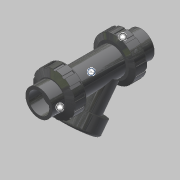
# Autodesk Inventor part: STRAINER Y-TYPE GLUED DN40
Saved by Autodesk Inventor 2017 (Build 210142000, 142)
## iProperties
Company: Pocket Brewery Belgium
Created: 2016-04-26
Part Number: STRAINER Y-TYPE GLUED DN40
Description: RVUIV VINK
Document SubType Name: Modeling
Manufacturer: SEKISUI
Mass: 197.859 g
Surface Area: 285.44 cm^2
Volume: 153.379 cm^3
Density: 1.29 g/cm^3
Material: U-PVC
Appearance: Smooth - Medium Gray
Catalog Web Link: http://www.pocketbrewery.com
Title: BALL VALVE PVC-U TRD DN15
Autodesk Inventor part; units mm, degrees
ref_plane "YZ Plane" through (0, 0, 0) normal (1, 0, 0) x (0, 1, 0)
ref_plane "XZ Plane" through (0, 0, 0) normal (0, 1, 0) x (-1, 0, 0)
ref_plane "XY Plane" through (0, 0, 0) normal (0, 0, 1) x (1, 0, 0)
sketch "Sketch_1" plane through (0, 0, 0) normal (1, 0, 0) x (0, 1, 0)
  line L0 (90.5, 0) -> (90.5, -33.3333)
  line L1 (90.5, -33.3333) -> (84.4338, -50)
  line L2 (84.4338, -50) -> (58.7082, -50)
  line L3 (58.7082, -50) -> (54.3, -37.8886)
  line L4 (54.3, -37.8886) -> (54.3, -25)
  line L5 (-54.3, -25) -> (-54.3, -37.8886)
  line L6 (-54.3, -37.8886) -> (-58.7082, -50)
  line L7 (-58.7082, -50) -> (-84.4338, -50)
  line L8 (-84.4338, -50) -> (-90.5, -33.3333)
  line L9 (-90.5, -33.3333) -> (-90.5, 0)
  line L10 (-90.5, 0) -> (90.5, 0)
  line L11 (-58.7082, -50) -> (0, -50) construction
  line L12 (0, -50) -> (0, -44.4444) construction
  line L13 (-85.1618, -50) -> (-60.7082, -50)
  line L14 (-60.7082, -50) -> (-60.7082, -48)
  line L15 (-60.7082, -48) -> (-85.1618, -48)
  line L16 (-85.1618, -48) -> (-85.1618, -50)
  line L17 (60.7082, -50) -> (85.1618, -50)
  line L18 (85.1618, -50) -> (85.1618, -48)
  line L19 (85.1618, -48) -> (60.7082, -48)
  line L20 (60.7082, -48) -> (60.7082, -50)
  line L21 (-54.3, -25) -> (54.3, -25)
  point P0 (0, 0)
  point P1 (0, 0)
  point P2 (-71.571, -50)
  point P3 (0, 0)
  dimension "dimZ" = 181
  dimension "dimE" = 100
  dimension "d22" = 50
  dimension "d23" = 16.6667
  dimension "d24" = 20
  dimension "d27" = 36.2
  dimension "d28" = 36.2
  dimension "d40" = 5.5556
  dimension "d52" = 20
  dimension "d53" = 2
  dimension "d54" = 2
  dimension "d55" = 2
  dimension "d73" = 50
  dimension "d74" = 16.6667
  constraints: 44 end point, 6 parallel, 5 equal length, 5 horizontal, 5 perpendicular, 4 point on line, 3 collinear, 2 coincident, 2 midpoint
  measures "dimZ" distance of L9.end L0.start
  measures "dimE" diameter of L2 L10
  measures "d22" distance from line of L0.start L2
  measures "d23" vertical distance of L1.start L1.end
  measures "d24" angle of L0 L1
  measures "d27" distance between parallel lines of L9 L5
  measures "d28" distance between parallel lines of L0 L4
  measures "d40" distance of L11.end L12.end
  measures "d52" angle of L5 L6
  measures "d53" distance of L15.end L13.start
  measures "d54" distance from line of L6.end L14
  measures "d55" distance from line of L2.end L20
  measures "d73" diameter of L21 L10
  measures "d74" distance from line of L8.end L7
revolve "Revolution1" add sketch "Sketch_1" angle 360 about axis through (0, -90.5, 0) along (0, 1, 0) contours L0 L1 L19 L20 L2 L3 L4 L21 L5 L6 L7 L14 L15 L8 L9 L10 | L1 L2 L20 L19 | L15 L14 L7 L8 | L8 L13 L16
sketch "Sketch_7" plane through (0, 0, 0) normal (1, 0, 0) x (0, 1, 0)
  line L0 (-121.5, 31.5) -> (121.5, 31.5)
  line L1 (121.5, 0) -> (-121.5, 0)
  line L2 (-121.5, 31.5) -> (-121.5, 25)
  line L3 (-121.5, 25) -> (121.5, 25)
  line L4 (121.5, 25) -> (121.5, 31.5)
  point P0 (0, 0)
  point P1 (0, 0)
  point P2 (0, 0)
  dimension "dimH" = 243
  dimension "dimD" = 50
  dimension "dimD2" = 63
  constraints: 10 end point, 2 coincident, 2 perpendicular, 2 point on line, 1 horizontal, 1 midpoint, 1 parallel, 1 vertical
  measures "dimH" distance of L2.end L3.end
  measures "dimD" diameter of L3 L1
  measures "dimD2" diameter of L0 L1
revolve "Revolution3" add sketch "Sketch_7" angle 360 about axis through (0, 121.5, 0) along (0, -1, 0)
extrude "Extrusion8" cut sketch "Sketch_1" along normal mid plane 6.6667 contours L18 L17 L1 | L1 L2 L20 L19 | L15 L14 L7 L8 | L8 L13 L16
pattern_circular "Circular Pattern1" count 14 over 360 about axis through (0, 0, 0) along (0, -1, 0) of "Extrusion8"
sketch "Sketch16" plane through (0, 0, 0) normal (1, 0, 0) x (0, 1, 0)
  line L0 (-54.3, -31.5) -> (7.4239, -112.3544)
  line L1 (7.4239, -112.3544) -> (32.462, -93.2404)
  line L2 (32.462, -93.2404) -> (-29.2619, -12.386)
  line L3 (-29.2619, -12.386) -> (-54.3, -31.5)
  line L4 (-29.2619, -12.386) -> (-4.2238, 6.728) construction
  line L5 (-4.2238, 6.728) -> (57.5001, -74.1265) construction
  line L6 (57.5001, -74.1265) -> (32.462, -93.2404) construction
  line L7 (7.4239, -112.3544) -> (-2.5913, -120)
  line L8 (-2.5913, -120) -> (-23.829, -92.1799)
  line L9 (-23.829, -92.1799) -> (-13.8138, -84.5343)
  line L10 (57.5001, -74.1265) -> (67.5153, -66.4809) construction
  line L11 (67.5153, -66.4809) -> (46.2776, -38.6608) construction
  line L12 (46.2776, -38.6608) -> (36.2624, -46.3064) construction
  line L13 (0, -178.6) -> (0, 98.6) projected
  line L14 (-95.6245, 0) -> (107.5467, 0) projected
  line L15 (54.3, -31.5) -> (-54.3, -31.5) projected
  line L16 (58.7082, -50) -> (58.7082, 50) projected
  point P0 (3.8866, 0)
  dimension "d75" = 63
  dimension "d77" = 12.6
  dimension "d78" = 35
  dimension "d80" = 120
  dimension "d83" = 3
  constraints: 26 end point, 10 perpendicular, 5 equal length, 3 point on line
  measures "d75" distance between parallel lines of L5 L0
  measures "d77" distance of L0.end L7.end
  measures "d78" distance of L7.end L8.end
  measures "d80" vertical distance of L7.end point (3.887, 0)
  measures "d83" distance from line of L16.start L11
revolve "Revolution7" add sketch "Sketch16" angle 360 about axis through (0, 32.462, -93.2404) along (0, -0.606793, 0.7948599) contours L15 L2 L13 L0 | L3 L2 L15 | L0 L13 L7 L8 L9 | L13 L2 L1 L0 | L0 L7 L13
fillet "Fillet2" radius 5 1 edges at (0, 67.5153, -66.4809)
equation "\"d23\" = 0.333333 * d22"
equation "\"d28\" = d27"
equation "\"d40\" = 0.333333 * d23"
equation "\"d47\" = 0.0666667 * dimE"
body "Solid1"
